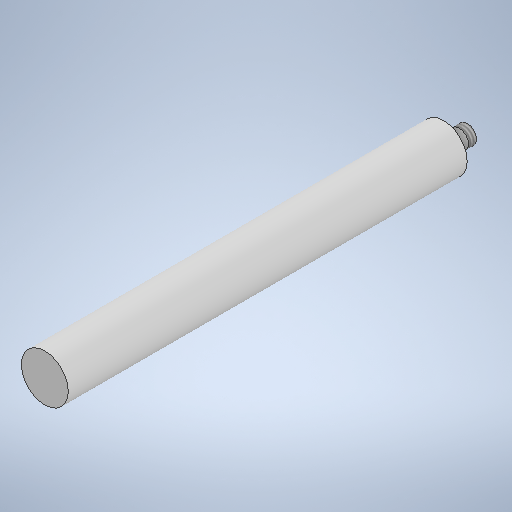
# Autodesk Inventor part: TS_V1_Fallmagazin_Blech_int
Saved by Autodesk Inventor 2025.2 (Build 292293000, 293)
## iProperties
Created: 2025-06-13
Part Number: TS_V1_Fallmagazin_Blech_int
Material: Generisch
Document SubType Name: Modeling
Designer: tino
Density: 1 g/cm^3
Appearance: Vorgabe
Author: tino
Autodesk Inventor part; units mm, degrees
ref_plane "YZ Plane" through (0, 0, 0) normal (1, 0, 0) x (0, 1, 0)
ref_plane "XZ Plane" through (0, 0, 0) normal (0, 1, 0) x (-1, 0, 0)
ref_plane "XY Plane" through (0, 0, 0) normal (0, 0, 1) x (1, 0, 0)
sketch "Skizze6" plane through (0, 0, 0) normal (1, 0, 0) x (0, 1, 0)
  line L0 (-253.2103, 0) -> (-253.2103, 5)
  line L1 (-253.2103, 5) -> (-168.2103, 5)
  line L2 (-168.2103, 5) -> (-168.2103, 1.6557)
  line L3 (-168.2103, 1.6557) -> (-166.2103, 1.6557)
  line L4 (-166.2103, 1.6557) -> (-164.9254, 2)
  line L5 (-164.9254, 2) -> (-163.2103, 2)
  line L6 (-163.2103, 2) -> (-163.2103, 0)
  line L7 (-163.2103, 0) -> (-253.2103, 0)
  point P0 (0, 0)
  dimension "d31" = 5
  dimension "d32" = 85
  dimension "d33" = 5
  dimension "d34" = 2
  dimension "d35" = 15
  dimension "d36" = 2
  constraints: 16 end point, 5 perpendicular, 1 parallel, 1 vertical
  measures "d31" distance of L0.start L0.end
  measures "d32" distance of L0.end L1.end
  measures "d33" distance between parallel lines of L2 L6
  measures "d34" distance of L2.end L3.end
  measures "d35" angle of L3 L4
  measures "d36" distance of L5.end L6.end
revolve "Umdrehung1" add sketch "Skizze6" angle 360 about axis through (0, -163.2103, 0) along (0, -1, 0)
thread "Gewinde2" size "M4x0.7" class "6g" standard "ANSI Metric M Profile" full length
fillet "Rundung6" radius 0.4 2 edges at (0, -166.2103, -1.6557) (0, -168.2103, -1.6557)
